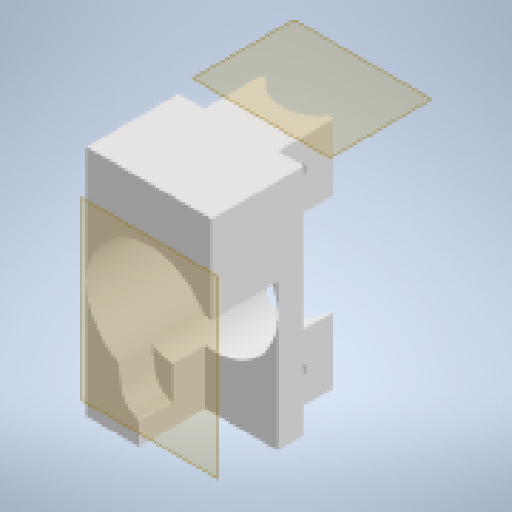
# Autodesk Inventor part: Servo Mount V4
Saved by Autodesk Inventor 2024 (Build 280153000, 153)
## iProperties
Created: 2024-11-24
Part Number: Servo Mount V4
Material: Generic
Document SubType Name: Modeling
Designer: Tommy Rohmann
Density: 1 g/cm^3
Appearance: Default
Author: Tommy Rohmann
Autodesk Inventor part; units mm, degrees
ref_plane "YZ Plane" through (0, 0, 0) normal (1, 0, 0) x (0, 1, 0)
sketch "Servo Containment" plane through (0, 0, 0) normal (0, 0, 1) x (1, 0, 0)
  line L0 (-22.2827, 48.831) -> (-35.4907, 48.831)
  line L1 (-35.4907, 48.831) -> (-35.4907, 18.351)
  line L2 (-35.4907, 18.351) -> (-22.2827, 18.351)
  line L3 (-22.2827, 18.351) -> (-22.2827, 48.831)
  line L4 (-22.2827, 45.275) -> (-35.4907, 45.275)
  line L5 (-35.4907, 45.275) -> (-35.4907, 21.907)
  line L6 (-35.4907, 21.907) -> (-22.2827, 21.907)
  line L7 (-22.2827, 21.907) -> (-22.2827, 45.275)
  line L8 (-28.8867, 18.351) -> (-28.8867, 21.907) construction
  line L9 (-28.8867, 45.275) -> (-28.8867, 48.831) construction
  line L10 (-28.8867, 21.907) -> (-28.8867, 27.749)
  point P0 (-28.8867, 33.0211)
  dimension "d0" = 13.208
  dimension "d1" = 30.48
  dimension "d2" = 23.368
  dimension "d4" = 5.842
  measures "d0" distance of L2.end L1.end
  measures "d1" distance of L1.end L0.end
  measures "d2" distance of L5.end L4.end
  measures "d4" distance of L8.end L10.end
sketch "zdstj" plane through (0, 0, 0) normal (0, 0, 1) x (1, 0, 0)
  line L0 (-10.4838, -7.9303) -> (-9.9261, -12.0195)
  arc A0 (-9.9261, -12.0195) -> (1.399, -12.0195) centre (-4.2636, -11.2472) ccw
  point P0 (-6.5265, -10.9007)
ref_plane "Work Plane1" through (0, 0, 0) normal (0, 0, 1) x (1, 0, 0)
sketch "Sketch1" plane through (0, 0, 0) normal (0, 0, 1) x (1, 0, 0)
  arc A0 (6.2203, -7.2241) -> (-6.2203, -7.2241) centre (0, 3.556) ccw projected
  line L0 (2.032, 8.0666) -> (2.032, -8.723) projected
  arc A1 (4.826, -6.5243) -> (4.826, 13.6363) centre (0, 3.556) ccw projected
  arc A2 (2.032, -8.723) -> (-2.032, -8.723) centre (0, 3.556) ccw projected
  line L1 (-12.7635, 27.3431) -> (12.7635, 27.3431)
  line L2 (12.7635, 27.3431) -> (12.7635, -20.2311)
  line L3 (12.7635, -20.2311) -> (-12.7635, -20.2311)
  line L4 (-12.7635, -20.2311) -> (-12.7635, 27.3431)
  arc A3 (-5.6626, -11.3133) -> (5.6626, -11.3133) centre (0, -10.541) ccw projected
  line L5 (-6.2203, -7.2241) -> (-5.6626, -11.3133) projected
  line L6 (-6.2203, -7.2241) -> (-6.2203, -20.2311)
  circle A4 centre (0, 3.556) radius 12.7635
  line L7 (14.097, 3.556) -> (0, 3.556)
  line L8 (6.604, 24.638) -> (-6.604, 24.638)
  line L9 (-6.604, 24.638) -> (-6.604, -5.842)
  line L10 (-6.604, -5.842) -> (6.604, -5.842)
  line L11 (6.604, -5.842) -> (6.604, 24.638)
  line L12 (6.604, 21.082) -> (-6.604, 21.082)
  line L13 (-6.604, 21.082) -> (-6.604, -2.286)
  line L14 (-6.604, -2.286) -> (6.604, -2.286)
  line L15 (6.604, -2.286) -> (6.604, 21.082)
  line L16 (0, -5.842) -> (0, -2.286) construction
  line L17 (0, 21.082) -> (0, 24.638) construction
  line L18 (0, -2.286) -> (0, 3.556)
  line L19 (10.7801, 9.7763) -> (14.8693, 9.2186)
  arc A5 (14.8693, 9.2186) -> (14.8693, -2.1066) centre (14.097, 3.556) cw
  point P0 (0, 0)
  point P1 (0, 3.556)
  point P2 (0, -19.05)
  point P3 (12.7635, 27.3431)
  point P4 (-12.7635, -20.2311)
  point P5 (6.604, 14.4782)
  point P6 (11.1751, 9.7224)
  point P7 (12.7635, 9.5058)
  point P8 (-12.7635, 3.556)
  point P9 (-6.604, 14.4782)
  point P10 (-6.604, 14.1054)
  point P11 (6.604, 14.1054)
  point P12 (-6.2203, -7.5892)
  constraints: 12 end point, 2 horizontal, 2 parallel, 2 perpendicular, 1 centre point, 1 coincident, 1 point on line, 1 tangent, 1 vertical, 5 other
ref_plane "Work Plane2" through (-12.7635, 27.3431, -23.876) normal (0, 1, 0) x (1, 0, 0)
sketch "Sketch2" plane through (-12.7635, 27.3431, -23.876) normal (0, 1, 0) x (1, 0, 0)
  arc A0 (17.5895, 10.6426) -> (7.9375, 10.6426) centre (12.7635, 10.6426) ccw projected
  line L0 (17.5895, 0) -> (17.5895, 10.6426) projected
  line L1 (7.9375, 10.6426) -> (7.9375, 0) projected
  arc A1 (20.2819, 10.6426) -> (5.2451, 10.6426) centre (12.7635, 10.6426) ccw projected
  line L2 (20.2819, 10.6426) -> (20.2819, 0) projected
  line L3 (20.2819, 10.6426) -> (20.2819, 0) projected
  line L4 (25.527, -5.08) -> (25.527, 18.796) projected
  line L5 (0, 18.796) -> (25.527, 18.796) projected
  line L6 (0, -5.08) -> (0, 18.796) projected
  line L7 (5.2451, 0) -> (5.2451, 10.6426) projected
  arc A2 (20.2819, 10.6426) -> (5.2451, 10.6426) centre (12.7635, 10.6426) ccw projected
  circle A3 centre (12.7635, 10.6426) radius 7.5184
  line L8 (20.2819, 0) -> (20.32, 0) projected
  line L9 (20.32, 0) -> (20.32, -5.08) projected
  line L10 (25.527, -5.08) -> (20.32, -5.08) projected
  line L11 (5.207, -5.08) -> (0, -5.08) projected
  line L12 (5.207, 0) -> (5.207, -5.08) projected
  line L13 (5.207, 0) -> (5.2451, 0) projected
  line L14 (5.207, -5.08) -> (20.32, -5.08)
  line L15 (20.2819, 0) -> (20.2819, -5.08)
  line L16 (5.2451, 0) -> (5.2451, -5.08)
  point P0 (12.7635, -23.876)
  point P1 (20.2819, 10.6426)
  point P2 (5.2451, 10.6426)
  constraints: 6 end point, 2 perpendicular, 2 point on line, 1 centre point, 1 coincident, 1 concentric, 1 horizontal
ref_plane "Work Plane3" through (-12.7635, -20.2311, -42.672) normal (0, -1, 0) x (1, 0, 0)
extrude "Extrusion1" add sketch "Sketch2" against normal up to surface (47.5742 mm away) contours A3 L2 L15 L14 L16 L7
fillet "Fillet1" radius 0.762 2 edges at (-7.5184, 3.556, -34.5186) (7.5184, 3.556, -34.5186)
extrude "Extrusion2" add sketch "Sketch1" against normal up to surface (18.796 mm away) contours A4 L11 L8 L9 L4 L1 L2 L19 | A4 L9 L12 L11 | L3 L4 A4 L6 | L12 L9 L8 L11
sketch "Sketch3" plane through (-7.5184, -20.2311, -23.876) normal (-1, 0, 0) x (0, 0, 1)
  circle A0 centre (0.9779, 6.1087) radius 1.6637 projected
  circle A1 centre (0.9779, 41.4655) radius 1.6637 projected
  point P0 (23.876, 20.2311)
extrude "Extrusion3" cut sketch "Sketch3" against normal blind 25.4
sketch "Sketch7" plane through (0, 3.556, -18.796) normal (0, 0, 1) x (1, 0, 0)
  circle A0 centre (0, 0) radius 12.7635 projected
  line L0 (12.7635, 23.7871) -> (12.7635, -23.7871) projected
  line L1 (12.7635, -23.7871) -> (-12.7635, -23.7871) projected
  line L2 (-12.7635, 23.7871) -> (12.7635, 23.7871) projected
  line L3 (-12.7635, -23.7871) -> (-12.7635, 23.7871) projected
  line L4 (-6.2203, -11.1452) -> (-6.2203, -23.7871) projected
  arc A1 (-5.6626, -14.8693) -> (5.6626, -14.8693) centre (0, -14.097) ccw projected
  line L5 (-6.2203, -10.7801) -> (-5.6626, -14.8693) projected
  line L6 (-2.032, -23.7871) -> (-2.032, 22.087)
  line L7 (0, -23.7871) -> (0, 23.7871)
  line L8 (12.7635, 5.9498) -> (11.1751, 6.1664) projected
  point P0 (0, -3.556)
  point P1 (-2.032, -19.4386)
  point P2 (-6.1664, -11.1751)
  point P3 (12.7635, 0)
  point P4 (-2.032, -12.6007)
  dimension "d17" = 2.032
  constraints: 4 end point, 2 midpoint, 1 point on line, 1 vertical
  measures "d17" distance between parallel lines of L6 L7
extrude "Extrusion4" add sketch "Sketch7" along normal blind 5.334 contours L0 L1 L7 A0 | A0 L8 L0 | L7 A1 L6 A0 | L6 A1 L5 A0 | L7 L1 L6 A1 | L5 A1 L6 L1 L4 A0
extrude "Extrusion5" add sketch "Sketch7" along normal up to surface (18.796 mm away) contours L5 A1 L6 L1 L4 A0
extrude "Extrusion6" cut sketch "Sketch7" along normal mid plane 55.5625 contours A0 L7 | A0 L6 L7 | A0 L6
ref_plane "Work Plane4" through (-6.2203, -16.256, -6.731) normal (0, 0, -1) x (0, 1, 0)
extrude "Extrusion7" add sketch "Sketch7" along normal up to surface (12.065 mm away) contours L6 A1 L5 A0
ref_plane "Work Plane5" through (0, 0, 9.144) normal (0, 0, 1) x (1, 0, 0)
sketch "Sketch14" plane through (0, 0, 9.144) normal (0, 0, 1) x (1, 0, 0)
  line L0 (-12.7635, -20.2311) -> (-12.7635, 27.3431) projected
  line L1 (12.7635, 27.3431) -> (-12.7635, 27.3431) projected
  line L2 (12.7635, 27.3431) -> (12.7635, -20.2311) projected
  line L3 (12.7635, -20.2311) -> (-12.7635, -20.2311) projected
  line L4 (-6.604, 24.638) -> (-6.604, -5.842) projected
  line L5 (-6.604, -5.842) -> (6.604, -5.842) projected
  line L6 (6.604, -5.842) -> (6.604, 24.638) projected
  line L7 (6.604, 24.638) -> (-6.604, 24.638) projected
  line L8 (6.604, 21.082) -> (-6.604, 21.082) projected
  line L9 (-6.604, -2.286) -> (6.604, -2.286) projected
  arc A0 (11.1751, 9.7224) -> (-12.7635, 3.556) centre (0, 3.556) ccw projected
  line L10 (0, 16.3195) -> (12.7635, 16.3195)
  arc A1 (-2.032, -9.0447) -> (12.7635, 3.556) centre (0, 3.556) ccw projected
  line L11 (0, -9.2075) -> (12.7635, -9.2075)
  point P0 (0, 0)
  constraints: 4 end point, 2 perpendicular, 2 point on circle, 2 point on line, 2 tangent
extrude "Extrusion8" add sketch "Sketch14" against normal up to surface (9.144 mm away) contours L0 A0 L4 L5 L6 L10 L2 A1 L11 L3 | L0 L1 L2 L10 L6 L7 L4 A0 | L11 A1 L2
extrude "Extrusion9" add sketch "Sketch14" along normal blind 3.175 contours L0 A0 L4 L5 L6 L10 L2 A1 L11 L3 | L0 L1 L2 L10 L6 L7 L4 A0 | L11 A1 L2 | L4 L7 L6 L8 | L9 L6 L5 L4
extrude "Extrusion10" cut sketch "Sketch14" against normal up to surface (22.606 mm away) contours A0 L6 L9 L4 | L4 L8 L6 L10 A0 | L4 L7 L6 L8 | L10 L6 A0
sketch "Sketch15" plane through (0, 3.556, -18.796) normal (0, 0, -1) x (-1, 0, 0)
  line L0 (0, -12.7635) -> (-22.033, -12.7635)
  line L1 (-22.033, -12.7635) -> (-22.033, 12.7635)
  line L2 (0, 12.7635) -> (-22.033, 12.7635)
  line L3 (-22.033, -12.7635) -> (27.2623, -12.7635)
  line L4 (27.2623, -12.7635) -> (27.2623, 12.7635)
  line L5 (27.2623, 12.7635) -> (-22.033, 12.7635)
  line L6 (-22.033, 12.7635) -> (-22.033, -12.7635)
  point P0 (0, -3.556)
  point P1 (0, -12.7635)
  constraints: 14 end point, 3 perpendicular, 2 horizontal, 2 parallel, 4 other
extrude "Extrusion11" cut sketch "Sketch15" along normal blind 14.2875 and the other way blind 19.0627
body "Solid1"
